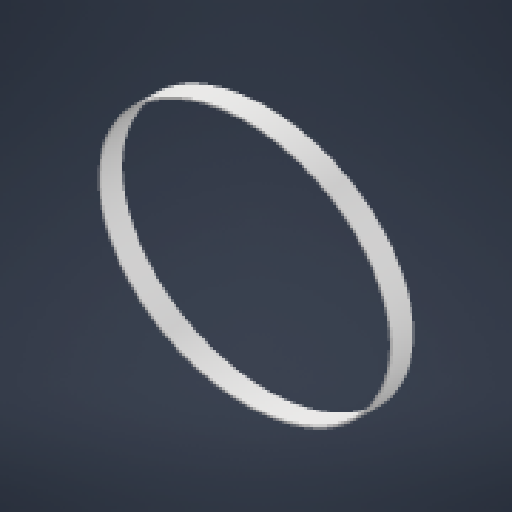
# Autodesk Inventor part: mounting_ring
Saved by Autodesk Inventor 2024 (Build 280153000, 153)
## iProperties
Created: 2026-08-20
Part Number: mounting_ring
Material: Generic
Document SubType Name: Modeling
Designer: schar
Density: 1 g/cm^3
Appearance: Default
Author: schar
Autodesk Inventor part; units mm, degrees
ref_plane "YZ Plane" through (0, 0, 0) normal (1, 0, 0) x (0, 1, 0)
ref_plane "XZ Plane" through (0, 0, 0) normal (0, 1, 0) x (-1, 0, 0)
ref_plane "XY Plane" through (0, 0, 0) normal (0, 0, 1) x (1, 0, 0)
sketch "Sketch1" plane through (0, 0, 0) normal (0, 0, 1) x (1, 0, 0)
  line L0 (0, 0) -> (0, 31) projected
  line L1 (0, 15.5) -> (-120, 15.5)
  ellipse E0 centre (-120, 15.5) end of major axis (0, 15.5) minor radius 101.3029
  ellipse E1 centre (-120, 15.5) end of major axis (-1.7, 15.5) minor radius 99.6029
  dimension "d0" = 120
  constraints: 2 end point, 2 horizontal, 1 centre point, 1 coincident, 1 horizontal alignment, 1 midpoint, 2 other
  measures "d0" distance of L1.start L1.end
extrude "Extrusion1" add sketch "Sketch1" against normal blind 18
body "Solid1"
